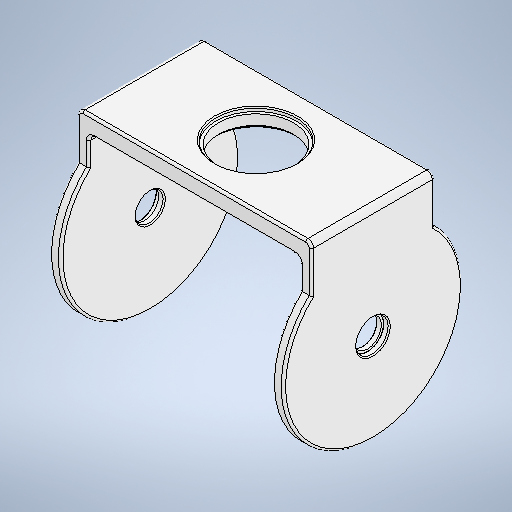
# Autodesk Inventor part: joint4_frame
Saved by Autodesk Inventor 2025.3 (Build 293356030, 356C)
## iProperties
Created: 2025-08-30
Part Number: joint4_frame
Material: PLA filament
Document SubType Name: Modeling
Designer: MSI
Density: 1.2 g/cm^3
Appearance: 일반
Mass: 862.584 g
Surface Area: 1402.45 cm^2
Volume: 718.82 cm^3
Author: MSI
Autodesk Inventor part; units mm, degrees
ref_plane "YZ Plane" through (0, 0, 0) normal (1, 0, 0) x (0, 1, 0)
ref_plane "XZ Plane" through (0, 0, 0) normal (0, 1, 0) x (-1, 0, 0)
ref_plane "XY Plane" through (0, 0, 0) normal (0, 0, 1) x (1, 0, 0)
sketch "스케치1" plane through (0, 0, 0) normal (1, 0, 0) x (0, 1, 0)
  circle A0 centre (0, 0) radius 80
  line L0 (0, 55) -> (99.7, 55)
  line L1 (99.7, 55) -> (99.7, -55)
  line L2 (99.7, -55) -> (0, -55)
  line L3 (0, -55) -> (0, 55)
  point P0 (58.0948, -55)
  point P1 (58.0948, 55)
  dimension "d0" = 160
  dimension "d1" = 99.7
  dimension "d36" = 110
  constraints: 8 end point, 3 coincident, 2 parallel, 1 centre point, 1 horizontal, 1 midpoint, 1 perpendicular
  measures "d0" diameter of A0
  measures "d1" distance of L1.end L2.end
  measures "d36" distance of L0.end L1.end
extrude "돌출1" add sketch "스케치1" along normal mid plane 209
sketch "스케치2" plane through (-104.5, 0, 55) normal (0, 0, 1) x (1, 0, 0)
  line L0 (10, 83.7) -> (199, 83.7)
  line L1 (199, 83.7) -> (199, -166.3)
  line L2 (199, -166.3) -> (10, -166.3)
  line L3 (10, -166.3) -> (10, 83.7)
  line L4 (209, 99.7) -> (0, 99.7) projected
  line L5 (0, 58.0948) -> (0, 99.7) projected
  point P0 (104.5, 0)
  point P1 (104.5, 0)
  point P2 (104.5, 83.7)
  dimension "d4" = 16
  dimension "d5" = 10
  dimension "d37" = 250
  constraints: 8 end point, 2 parallel, 1 coincident, 1 horizontal, 1 midpoint, 1 perpendicular, 1 vertical alignment
  measures "d4" distance between parallel lines of L0 L4
  measures "d5" distance between parallel lines of L5 L3
  measures "d37" distance of L2.end L0.start
extrude "돌출2" cut sketch "스케치2" along normal through all both and the other way through all
sketch "스케치4" plane through (-104.5, 99.7, 55) normal (0, 1, 0) x (1, 0, 0)
  point P0 (104.5, 55)
  point P1 (104.5, 55)
  constraints: 1 coincident
hole "구멍1" at (0, 99.7, 0) direction (0, -1, 0) diameter 67 end through all counterbore diameter 72 counterbore depth 3.5
sketch "스케치7" plane through (-94.5, 83.7, 55) normal (0, -1, 0) x (1, 0, 0)
  circle A0 centre (94.5, -55) radius 33.5 projected
  point P0 (94.5, -55)
  constraints: 1 coincident
hole "구멍4" at (0, 83.7, 0) direction (0, 1, 0) diameter 67 end through all counterbore diameter 72 counterbore depth 3.5
sketch "스케치5" plane through (104.5, 0, 0) normal (1, 0, 0) x (0, 0, -1)
  arc A0 (-55, 58.0948) -> (55, 58.0948) centre (0, 0) ccw projected
  point P0 (-80, 0)
  constraints: 1 coincident
hole "구멍2" at (104.5, 0, 0) direction (-1, 0, 0) diameter 25 end through all counterbore diameter 29 counterbore depth 5
mirror "미러1" about plane through (0, 0, 0) normal (1, 0, 0) of "구멍2"
fillet "모깎기1" radius 5 2 edges at (-94.5, 83.7, 0) (94.5, 83.7, 0)
fillet "모깎기2" radius 5 2 edges at (-104.5, 99.7, 0) (104.5, 99.7, 0)
fillet "모깎기3" radius 2 24 edges at (-93.0355, 82.2355, 55) (0, 83.7, 55) (93.0355, 82.2355, 55) (94.5, 68.3974, 55) (94.5, -80, 0) (94.5, 68.3974, -55) (93.0355, 82.2355, -55) (0, 83.7, -55) (-93.0355, 82.2355, -55) (-94.5, 68.3974, -55) (-94.5, -80, 0) (-94.5, 68.3974, 55) (104.5, -80, 0) (104.5, 76.3974, -55) (103.0355, 98.2355, -55) (0, 99.7, -55) (-103.0355, 98.2355, -55) (-104.5, 76.3974, -55) (-104.5, -80, 0) (-104.5, 76.3974, 55) (-103.0355, 98.2355, 55) (0, 99.7, 55) (103.0355, 98.2355, 55) (104.5, 76.3974, 55)
fillet "모깎기4" radius 0.1 2 edges at (99.5, 0, 14.5) (-99.5, 0, 14.5)
chamfer "모따기1" distance 1 angle 45 6 edges at (94.5, 0, 12.5) (-94.5, 0, 12.5) (0, 99.7, -36) (0, 83.7, 36) (104.5, 0, 14.5) (-104.5, 0, 14.5)
